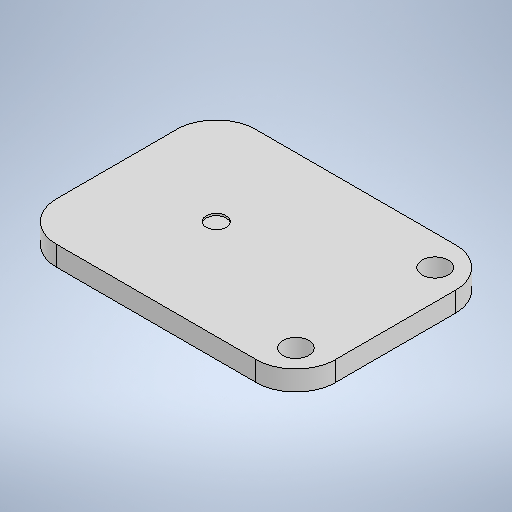
# Autodesk Inventor part: PNS-783 leg floor plate
Saved by Autodesk Inventor 2025 (Build 290162010, 162A)
## iProperties
Created: 2025-02-20
Part Number: PNS-783 leg floor plate
Material: Stainless Steel
Document SubType Name: Sheet Metal
Designer: admin
Mass: 1070.67 g
Surface Area: 320.872 cm^2
Volume: 133.833 cm^3
Density: 8 g/cm^3
Sheet Metal Rule: AISI304 3mm Die 32
Sheet Metal Width: 100,000 mm
Sheet Metal Length: 140,000 mm
Sheet Metal Area: 14000,000 mm^2
Appearance: Default
Flat Pattern Width: 10 cm
Flat Pattern Length: 14 cm
Flat Pattern Area: 140 cm^2
Author: user
Autodesk Inventor part; units mm, degrees
ref_plane "YZ Plane" through (0, 0, 0) normal (1, 0, 0) x (0, 1, 0)
ref_plane "XZ Plane" through (0, 0, 0) normal (0, 1, 0) x (-1, 0, 0)
ref_plane "XY Plane" through (0, 0, 0) normal (0, 0, 1) x (1, 0, 0)
sketch "Sketch1" plane through (0, 0, 0) normal (0, 0, 1) x (1, 0, 0)
  line L0 (-70, -50) -> (70, -50)
  line L1 (70, -50) -> (70, 50)
  line L2 (70, 50) -> (-70, 50)
  line L3 (-70, 50) -> (-70, -50)
  line L4 (-70, -50) -> (70, 50) construction
  line L5 (70, -50) -> (-70, 50) construction
  circle A0 centre (55, -35) radius 6.5
  circle A1 centre (55, 35) radius 6.5
  line L6 (0, 0) -> (70, 0) construction
  dimension "d0" = 140
  dimension "d1" = 100
  dimension "d23" = 13
  dimension "d25" = 15
  dimension "d26" = 15
  measures "d0" distance of L2.end L1.end
  measures "d1" distance of L1.end L0.end
  measures "d23" diameter of A0
  measures "d25" distance from line of L1 A0.centre
  measures "d26" distance from line of A0.centre L0
extrude "Plate1" add sketch "Sketch1" along normal blind 10
fillet "Corner Round1" radius 20 4 edges at (70, -50, 5) (-70, -50, 5) (-70, 50, 5) (70, 50, 5)
sketch "Sketch5" plane through (0, 0, 10) normal (0, 0, 1) x (1, 0, 0)
  line L0 (50, -50) -> (-50, -50) projected
  line L1 (-70, -30) -> (-70, 30) projected
  line L2 (-50, 50) -> (50, 50) projected
  circle A0 centre (-20, 0) radius 50
  circle A1 centre (-20, 0) radius 5
  point P0 (0, 0)
  dimension "d27" = 10
  constraints: 3 tangent, 2 centre point, 1 coincident
  measures "d27" diameter of A1
extrude "Extrusion2" cut sketch "Sketch5" against normal blind 1 contours A1
equation "\"d26\" = d25"
equation "\"d2\" = Thickness"
equation "\"BendReliefDepth\" = 0.5 * Thickness"
equation "\"TransitionRadius\" = BendRadius"
equation "\"JacobiRadiusSize\" = BendRadius"
equation "\"Thickness\" = 10"
equation "\"BendRadius\" = 5"
body "Solid1"
